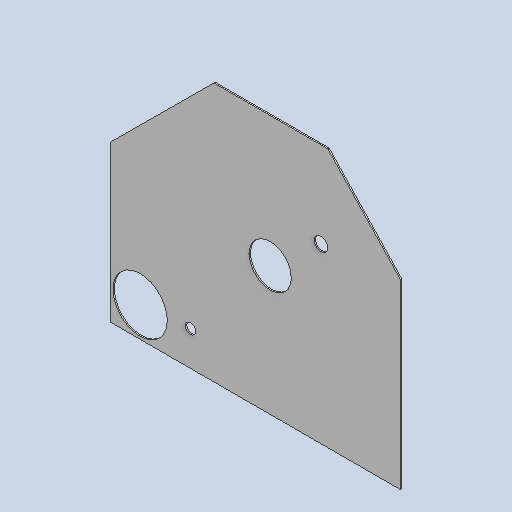
# Autodesk Inventor part: Left wall v2.0
Saved by Autodesk Inventor 2025 (Build 290162010, 162A)
## iProperties
Created: 2023-08-31
Part Number: Left wall v2.0
Material: Generic
Document SubType Name: Sheet Metal
Designer: admin
Density: 1 g/cm^3
Appearance: Default
Flat Pattern Width: 191 cm
Flat Pattern Length: 214 cm
Flat Pattern Area: 40874 cm^2
Sheet Metal Rule: Default
Sheet Metal Width: 1910,000 mm
Sheet Metal Length: 2140,000 mm
Sheet Metal Area: 4087400,000 mm^2
Stock Number: ДМФ 013 Стенка Нос
Author: admin
Autodesk Inventor part; units mm, degrees
ref_plane "YZ Plane" through (0, 0, 0) normal (1, 0, 0) x (0, 1, 0)
ref_plane "XZ Plane" through (0, 0, 0) normal (0, 1, 0) x (-1, 0, 0)
ref_plane "XY Plane" through (0, 0, 0) normal (0, 0, 1) x (1, 0, 0)
sketch "Sketch1" plane through (0, 0, 0) normal (0, 0, 1) x (1, 0, 0)
  line L0 (0, 0) -> (0, 1910) construction
  line L1 (424.5155, 1910) -> (-415.4845, 1910)
  line L2 (-415.4845, 1910) -> (-1180, 1150)
  line L3 (-1180, 0) -> (-1180, 1150)
  line L4 (960, 0) -> (960, 1342.8524)
  line L5 (424.5155, 1910) -> (960, 1342.8524)
  circle A0 centre (0, 950) radius 195 construction
  line L6 (960, 0) -> (-1180, 0)
  circle A1 centre (-960, 220) radius 200.5
  circle A2 centre (-588, 255) radius 38
  circle A3 centre (374.6358, 1277) radius 50
  circle A4 centre (0, 950) radius 155
  point P0 (0, 955)
  dimension "d1" = 840
  dimension "d3" = 1150
  dimension "d11" = 390
  dimension "d12" = 1180
  dimension "d13" = 950
  dimension "d14" = 76
  dimension "d15" = 1910
  dimension "d16" = 255
  dimension "d17" = 220
  dimension "d18" = 401
  dimension "d19" = 220
  dimension "d21" = 1277
  dimension "d22" = 1554.6358
  dimension "d23" = 100
  dimension "d33" = 2140
  dimension "d34" = 494
  dimension "d45" = 310
  dimension "d49" = 372
  dimension "d51" = 780
  dimension "d52" = 1078
  constraints: 14 end point, 5 centre point, 3 point on line, 3 vertical, 2 horizontal, 1 midpoint
  measures "d1" distance of L1.start L1.end
  measures "d3" distance of L3.start L2.end
  measures "d11" diameter of A0
  measures "d12" distance from line of L3 A0.centre
  measures "d13" distance from line of L6 A0.centre
  measures "d14" diameter of A2
  measures "d15" vertical distance of L3.start L1.end
  measures "d16" distance from line of A2.centre L6
  measures "d17" distance from line of L3 A1.centre
  measures "d18" diameter of A1
  measures "d19" distance from line of A1.centre L6
  measures "d21" distance from line of A3.centre L6
  measures "d22" distance from line of L3 A3.centre
  measures "d23" diameter of A3
  measures "d33" distance of L4.start L3.start
  measures "d34" distance of point (0, 955) A3.centre
  measures "d45" diameter of A4
  measures "d49" horizontal distance of A1.centre A2.centre
  measures "d51" distance of L1.start L4.end
  measures "d52" distance of L1.end L2.end
extrude "Extrusion1" add sketch "Sketch1" along normal blind 10
sketch "Sketch3" plane through (0, 0, 10) normal (0, 0, 1) x (1, 0, 0)
  line L0 (-400, 950) -> (400, 950) construction
  circle A0 centre (0, 950) radius 155 projected
  circle A1 centre (155, 950) radius 2.5
  circle A2 centre (-155, 950) radius 2.5
  line L1 (132.7592, 870) -> (-132.7592, 870) construction
  circle A3 centre (132.7592, 870) radius 2.5
  circle A4 centre (-132.7592, 870) radius 2.5
  point P0 (0, 0)
  point P1 (-154.9798, 947.5001)
  point P2 (-154.9798, 952.4999)
  point P3 (154.9798, 947.5001)
  point P4 (154.9798, 952.4999)
  point P5 (134.0322, 872.1516)
  point P6 (131.4516, 867.8692)
  dimension "d47" = 5
  dimension "d48" = 80
  constraints: 4 centre point, 4 coincident, 4 end point, 4 point on circle, 3 equal radius, 2 horizontal, 2 point on line, 1 midpoint
  measures "d47" diameter of A2
  measures "d48" distance between parallel lines of L1 L0
extrude "Extrusion3" cut sketch "Sketch3" against normal through all contours A0 A1 | A0 A2 | A3 A0 | A4 A0 | A0 A4 picked at (155.7492, 949.3589) picked at (-155.8257, 950.101) picked at (133.5004, 869.6223)
equation "\"d17\" = d19"
body "Solid1"
